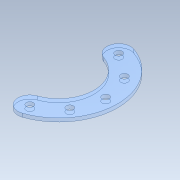
# Autodesk Inventor part: pulsador_presion
Saved by Autodesk Inventor 2022 (Build 260153000, 153)
## iProperties
Created: 2022-11-16
Part Number: pulsador_presion
Material: Generic
Document SubType Name: Modeling
Designer: ferna
Density: 1 g/cm^3
Appearance: Blue - Glazing
Author: ferna
Autodesk Inventor part; units mm, degrees
ref_plane "YZ Plane" through (0, 0, 0) normal (1, 0, 0) x (0, 1, 0)
ref_plane "XZ Plane" through (0, 0, 0) normal (0, 1, 0) x (-1, 0, 0)
ref_plane "XY Plane" through (0, 0, 0) normal (0, 0, 1) x (1, 0, 0)
sketch3d "3D Sketch1"
sketch "Sketch8" plane through (0, 0, 0) normal (0, 1, 0) x (-1, 0, 0)
  arc A0 (-533.9727, 129.2939) -> (-533.9727, 72.7061) centre (-524, 101) ccw projected
  arc A1 (-533.9727, 129.2939) -> (-540.6211, 148.1565) centre (-537.2969, 138.7252) ccw projected
  arc A2 (-540.6211, 148.1565) -> (-540.6211, 53.8435) centre (-524, 101) ccw projected
  arc A3 (-540.6211, 53.8435) -> (-533.9727, 72.7061) centre (-537.2969, 63.2748) ccw projected
  circle A4 centre (-537.2969, 63.2748) radius 3 projected
  circle A5 centre (-556.6482, 77.8001) radius 2.9994 projected
  circle A6 centre (-564, 101) radius 3 projected
  circle A7 centre (-556.6482, 124.1094) radius 2.9994 projected
  circle A8 centre (-537.2969, 138.7252) radius 3 projected
  point P0 (0, 0)
extrude "Extrusion1" add sketch "Sketch8" along normal blind 3
body "Solid1"
